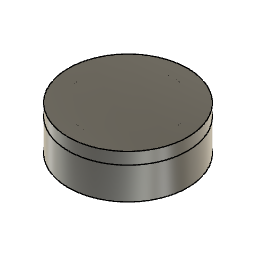
Zen_Garden_Model (Autodesk Fusion 360 design; units mm, degrees)
Autodesk Fusion 360 part; units mm, degrees
sketch "Sketch1" plane through (0, 0, 0) normal (0, 0, 1) x (1, 0, 0)
sketch "Sketch1 (2)" plane through (0, 0, 0) normal (0, 0, 1) x (1, 0, 0) in component "Base"
  circle A0 centre (0, 0) radius 120
  dimension "d2" = 240
  constraint coincident A0.centre origin
  measures "d2" diameter of A0
extrude "Extrude1" add sketch "Sketch1 (2)" along normal blind 10 makes body 1 in component "Base"
sketch "Sketch2" plane through (0, 0, 10) normal (0, 0, 1) x (-1, 0, 0) in component "Base"
  circle A0 centre (0, 0) radius 120
  circle A1 centre (0, 0) radius 100
  dimension "d5" = 20
  constraint coincident A0.centre A1.centre
  measures "d5" distance of A0 A1
extrude "Extrude2" add sketch "Sketch2" along normal blind 55 bodies 1 in component "Base"
sketch "Sketch3" plane through (0, 0, 65) normal (0, 0, 1) x (-1, 0, 0) in component "Base"
  circle A0 centre (0, 0) radius 100
  circle A1 centre (0, 0) radius 120
  circle A2 centre (0, 0) radius 107
  dimension "d10" = 7
  constraint coincident A0.centre A1.centre
  measures "d10" distance of A0 A2
extrude "Extrude3" add sketch "Sketch3" along normal blind 7 contours A1 bodies 1 in component "Base"
sketch "Sketch1 (3)" plane through (0, 0, 65) normal (0, 0, 1) x (-1, 0, 0) in component "Crown gear"
  circle A0 centre (0, 0) radius 73
  circle A1 centre (0, 0) radius 107
  circle A2 centre (0, 0) radius 107
  circle A3 centre (0, 0) radius 90 construction
  circle A4 centre (0, 0) radius 80
  circle A5 centre (0, 0) radius 100
  dimension "d92" = 180
  dimension "d164" = 7
  dimension "d168" = 7
  dimension "d170" = 10
  dimension "d171" = 10
  constraint coincident A0.centre A1.centre
  constraint equal A1 A2
  constraint concentric A2 A3
  constraint concentric A1 A4
  constraint concentric A1 A5
  measures "d92" diameter of A3
  measures "d164" distance of A1 A5
  measures "d168" distance of A0 A4
  measures "d170" distance of A3 A5
  measures "d171" distance of A3 A4
extrude "Extrude5" add sketch "Sketch1 (3)" against normal blind 15 separate body contours A1 A2 | A4 | A5 makes body 2 in component "Crown gear"
ref_plane "WorkPlane2" through (107, 0, 58.3628) normal (1, 0, 0) x (0, 1, 0) in component "Crown gear"
sketch "Sketch5" plane through (107, 0, 0) normal (1, 0, 0) x (0, 1, 0) in component "Crown gear"
  line L0 (-0.4478, 54) -> (-25.4478, 54) construction
  line L1 (-6.4157, 50) -> (-7.8716, 54)
  line L2 (-7.8716, 54) -> (-9.6915, 59)
  line L3 (-9.6915, 59) -> (0, 59)
  line L4 (0, 59) -> (-1.8199, 54)
  line L5 (-3.2757, 50) -> (-6.4157, 50)
  line L6 (-107, 50) -> (107, 50) construction
  line L7 (107, 65) -> (-107, 65) construction
  line L8 (-3.2757, 50) -> (-1.8199, 54)
  line L9 (0, 50) -> (0, 65) construction
  line L10 (3.2757, 50) -> (6.4157, 50)
  line L11 (6.4157, 50) -> (7.8716, 54)
  line L12 (0, 59) -> (1.8199, 54)
  line L13 (7.8716, 54) -> (9.6915, 59)
  line L14 (9.6915, 59) -> (0, 59)
  line L15 (3.2757, 50) -> (1.8199, 54)
  line L16 (3.2757, 50) -> (-3.2757, 50)
  point P0 (0, 50)
  point P1 (0.4478, 54)
  dimension "d102" = 70
  dimension "d103" = 70
  dimension "d104" = 4
  dimension "d105" = 5
  dimension "d107" = 3.14
  constraint horizontal L0
  constraint parallel L1 L2
  constraint parallel L0 L3
  constraint coincident L0 L4.end
  constraint horizontal L5
  constraint coincident L1.start L6
  constraint horizontal L0.start L1.end
  constraint equal L1 L8
  constraint midpoint L6 P0
  constraint midpoint L7 L9.end
  constraint vertical L3.end P0
  constraint symmetric L0.start L9 P1
  constraint symmetric L1.start L9 L10.end
  constraint symmetric L1.end L9 L11.end
  constraint symmetric L2.end L9 L13.end
  constraint symmetric L3.end L9 L4.start
  constraint symmetric L4.end L9 L12.end
  constraint symmetric L5.start L9 L10.start
  constraint symmetric P0 L9 L9.start
  measures "d102" angle of L0 L4
  measures "d103" angle of L0 L2
  measures "d104" vertical distance of L1.start L1.end
  measures "d105" vertical distance of L3.end L4.end
  measures "d107" distance of L1.start L5.start
extrude "Extrude6" cut sketch "Sketch5" along normal up to surface contours L4 L8 L12 L15 L16 end surface at (-72.6372, 7.2685, 55) on bodies 2 bodies 2 in component "Crown gear"
pattern_circular "C-Pattern2" count 45 over 360 about axis through (0, 0, 1.75) along (0, 0, 1) of "Extrude6" in component "Crown gear"
sketch "Sketch1 (4)" plane through (0, 0, 0) normal (1, 0, 0) x (0, 1, 0) in component "Pinion"
  circle A0 centre (0, 0) radius 20 construction
  circle A1 centre (0, 0) radius 20 construction
  circle A2 centre (0, 0) radius 18.7939
  circle A3 centre (0, 0) radius 24
  circle A4 centre (0, 0) radius 15
  line L0 (-18.7939, 0) -> (-18.7939, 29.5206) construction
  line L1 (0, 0) -> (-18.7939, 0) construction
  line L2 (0, 0) -> (-16.276, 9.3969) construction
  line L3 (0, 0) -> (-9.3969, 16.276) construction
  line L4 (0, 0) -> (0, 18.7939) construction
  line L5 (-16.276, 9.3969) -> (-6.4358, 26.4406) construction
  line L6 (-9.3969, 16.276) -> (-0.8751, 21.1961) construction
  spline S0 degree 5 poles (0, 18.7939) (0.0298, 18.9066) (0.0619, 19.1437) (0.0272, 19.5336) (-0.1787, 20.1207) (-0.672, 20.9554) (-1.3671, 21.8756) (-2.2385, 22.8636) (-3.2706, 23.8992) (-4.4543, 24.9586) (-5.7848, 26.0128) (-7.2591, 27.0265) (-8.8723, 27.9564) (-10.6168, 28.7521) (-12.485, 29.3613) (-14.4696, 29.7332) (-16.1459, 29.8058) (-17.4513, 29.7195) (-18.3428, 29.5976) (-18.7939, 29.5206) knots 0 0 0 0 0 0 0.066667 0.133333 0.2 0.266667 0.333333 0.4 0.466667 0.533333 0.6 0.666667 0.733333 0.8 0.866667 0.933333 1 1 1 1 1 1
  line L7 (0, 0) -> (-11.0467, 15.2045) construction
  line L8 (0, 18.7939) -> (-11.0467, 15.2045) construction
  line L9 (0, 0) -> (-5.5234, 16.9992) construction
  line L10 (0, 18.7939) -> (-5.5234, 16.9992) construction
  line L11 (0, 0) -> (-2.7617, 17.8965) construction
  spline S1 degree 5 poles (-5.6654, 17.9196) (-5.7278, 18.0181) (-5.8299, 18.2345) (-5.9144, 18.6168) (-5.895, 19.2386) (-5.6762, 20.1832) (-5.2909, 21.2701) (-4.7578, 22.4748) (-4.0859, 23.7734) (-3.2767, 25.1404) (-2.3258, 26.5465) (-1.2257, 27.9576) (0.0321, 29.3305) (1.4556, 30.6151) (3.0532, 31.759) (4.8334, 32.7119) (6.4098, 33.2865) (7.6805, 33.5977) (8.5673, 33.7502) (9.0206, 33.8128) knots 0 0 0 0 0 0 0.066667 0.133333 0.2 0.266667 0.333333 0.4 0.466667 0.533333 0.6 0.666667 0.733333 0.8 0.866667 0.933333 1 1 1 1 1 1
  line L12 (-0.4419, 17.1231) -> (0.4419, 20.4646)
  line L13 (-15.9559, 30.0052) -> (-21.6318, 29.036)
  line L14 (-4.7405, 16.4598) -> (-6.5903, 19.3794)
  line L15 (6.1687, 33.4193) -> (11.8726, 34.2062)
  point P0 (-5.5552, 20.4738)
  point P1 (-1.8342, 27.1507)
  dimension "d122" = 40
  dimension "d123" = 37.5877
  dimension "d124" = 48
  dimension "d125" = 30
  dimension "d126" = 29.5206
  dimension "d128" = -90
  dimension "d129" = 19.6804
  dimension "d130" = 9.8402
  dimension "d131" = 36
  constraint concentric A0 A1
  constraint concentric A0 A2
  constraint vertical A0.centre A1.centre
  constraint concentric A1 A3
  constraint concentric A2 A4
  constraint coincident A2 L0.start
  constraint tangent A2 L0
  constraint vertical L0
  constraint coincident A0.centre A1.centre
  constraint tangent A2 L5
  constraint perpendicular L2 L5
  constraint tangent A2 L6
  constraint perpendicular L3 L6
  constraint coincident A2 L7.end
  constraint midpoint L8 L9.end
  constraint midpoint L10 L11.end
  constraint midpoint L4.end L12
  constraint midpoint L0.end L13
  constraint symmetric L0.end L11 S1.end
  constraint symmetric L4.end L11 S1.start
  constraint symmetric L5.end L11 P1
  constraint symmetric L6.end L11 P0
  constraint symmetric L11 L12.start L14.start
  constraint symmetric L11 L12.end L14.end
  constraint symmetric L11 L13.start L15.start
  constraint symmetric L11 L13.end L15.end
  measures "d122" diameter of A0
  measures "d123" diameter of A2
  measures "d124" diameter of A3
  measures "d125" diameter of A4
  measures "d126" distance of L0.start L0.end
  measures "d129" distance of L2.end L5.end
  measures "d130" distance of L3.end L6.end
  measures "d131" angle of L4 L7
extrude "Extrude1'" add sketch "Sketch1 (4)" against normal blind 4 separate body contours A2 A3 S0 S1 picked at (-2.921, 21.0246) makes body 3 in component "Pinion"
pattern_circular "C-Pattern1" count 10 over 360 about axis through (1.75, 0, 0) along (1, 0, 0) of "Extrude1'" makes body 4 at (-0.3509, -16.7988, 14.2591) makes body 5 at (-0.3509, -21.9731, 1.6629) makes body 6 at (-0.3509, -18.755, -11.5701) makes body 7 at (-0.3509, -8.3701, -20.3829) makes body 8 at (-0.3509, 5.2072, -21.4147) makes body 9 at (-0.3509, 16.7988, -14.2591) makes body 10 at (-0.3509, 21.9731, -1.6629) makes body 11 at (-0.3509, 18.755, 11.5701) makes body 12 at (-0.3509, 8.3701, 20.3829) in component "Pinion"
extrude "Extrude2'" add sketch "Sketch1 (4)" against normal up to surface (4 mm away) contours A2 | A4 bodies 3 4 5 6 7 8 9 10 11 12 in component "Pinion"
sketch "Sketch8" plane through (0, 0, 0) normal (1, 0, 0) x (0, 1, 0) in component "Crown gear"
  line L0 (73, 59) -> (83, 59)
  line L1 (83, 59) -> (83, 50)
  line L2 (83, 50) -> (73, 50)
  line L3 (73, 50) -> (73, 59)
  line L4 (90, 65) -> (90, 50) construction
  line L5 (73, 65) -> (107, 65) construction
  line L6 (107, 50) -> (107, 59)
  line L7 (97, 50) -> (107, 50)
  line L8 (97, 59) -> (97, 50)
  line L9 (107, 59) -> (97, 59)
  point P0 (-73, 65)
  point P1 (73, 65)
  point P2 (107, 65)
  point P3 (-107, 65)
  point P4 (105.0137, 35)
  dimension "d139" = 9
  dimension "d140" = 10
  dimension "d172" = 6
  constraint horizontal L0
  constraint vertical L1
  constraint horizontal L2
  constraint vertical L3
  constraint vertical L4
  constraint coincident P1 L5.start
  constraint coincident P2 L5.end
  constraint midpoint L4.start L5
  constraint symmetric L0.start L4 L6.end
  constraint symmetric L0.end L4 L8.start
  constraint symmetric L1.end L4 L7.start
  constraint symmetric L4 L6.start L2.end
  constraint vertical P2 L6.start
  measures "d139" distance of L0.end L1.end
  measures "d140" distance of L0.start L0.end
  measures "d172" vertical distance of L0.start L5.start
revolve "Revolve2" cut sketch "Sketch8" angle 360 about axis through (0, 0, 1.75) along (0, 0, 1) bodies 2 in component "Crown gear"
sketch "Sketch2 (2)" plane through (0, 0, 0) normal (1, 0, 0) x (0, 1, 0) in component "Pinion"
  spline S0 degree 5 poles (17.874, 5.8076) (17.9905, 5.8141) (18.2258, 5.8569) (18.586, 6.0103) (19.0807, 6.3876) (19.7221, 7.1147) (20.3676, 8.0389) (20.8886, 8.9165) (21.274, 9.6386) (21.523, 10.1387) (21.6393, 10.3799) knots 0 0 0 0 0 0 0.066667 0.133333 0.2 0.266667 0.333333 0.392502 0.392502 0.392502 0.392502 0.392502 0.392502
  arc A0 (21.6393, 10.3799) -> (21.2067, 11.2372) centre (0, 0) ccw
  spline S1 degree 5 poles (15.2918, 10.9256) (15.3663, 11.0154) (15.5405, 11.1793) (15.878, 11.3778) (16.4753, 11.5516) (17.4413, 11.6354) (18.5681, 11.6054) (19.5836, 11.503) (20.3934, 11.3839) (20.9437, 11.2871) (21.2067, 11.2372) knots 0 0 0 0 0 0 0.066667 0.133333 0.2 0.266667 0.333333 0.392502 0.392502 0.392502 0.392502 0.392502 0.392502
  arc A1 (15.2918, 10.9256) -> (11.0467, 15.2045) centre (0, 0) ccw
  spline S2 degree 5 poles (11.0467, 15.2045) (11.1372, 15.2782) (11.3024, 15.4512) (11.5036, 15.787) (11.6821, 16.383) (11.7736, 17.3483) (11.7526, 18.4753) (11.6582, 19.4916) (11.5456, 20.3023) (11.4531, 20.8533) (11.4054, 21.1168) knots 0 0 0 0 0 0 0.066667 0.133333 0.2 0.266667 0.333333 0.392502 0.392502 0.392502 0.392502 0.392502 0.392502
  arc A2 (11.4054, 21.1168) -> (10.5515, 21.5561) centre (0, 0) ccw
  spline S3 degree 5 poles (5.9495, 17.8273) (5.9569, 17.9437) (6.0015, 18.1787) (6.1578, 18.5377) (6.539, 19.0294) (7.2712, 19.665) (8.2004, 20.3031) (9.0822, 20.8171) (9.8073, 21.1967) (10.3094, 21.4418) (10.5515, 21.5561) knots 0 0 0 0 0 0 0.066667 0.133333 0.2 0.266667 0.333333 0.392502 0.392502 0.392502 0.392502 0.392502 0.392502
  arc A3 (5.9495, 17.8273) -> (0, 18.7939) centre (0, 0) ccw
  spline S4 degree 5 poles (0, 18.7939) (0.0298, 18.9066) (0.0619, 19.1437) (0.0272, 19.5336) (-0.1787, 20.1207) (-0.672, 20.9554) (-1.3515, 21.8549) (-2.0252, 22.6216) (-2.5928, 23.2112) (-2.9915, 23.6027) (-3.185, 23.7877) knots 0 0 0 0 0 0 0.066667 0.133333 0.2 0.266667 0.333333 0.392502 0.392502 0.392502 0.392502 0.392502 0.392502
  arc A4 (-3.185, 23.7877) -> (-4.134, 23.6413) centre (0, 0) ccw
  spline S5 degree 5 poles (-5.6654, 17.9196) (-5.7278, 18.0181) (-5.8299, 18.2345) (-5.9144, 18.6168) (-5.895, 19.2386) (-5.6762, 20.1832) (-5.2995, 21.2456) (-4.8883, 22.1798) (-4.5249, 22.9131) (-4.2627, 23.4065) (-4.134, 23.6413) knots 0 0 0 0 0 0 0.066667 0.133333 0.2 0.266667 0.333333 0.392502 0.392502 0.392502 0.392502 0.392502 0.392502
  arc A5 (-5.6654, 17.9196) -> (-11.0467, 15.2045) centre (0, 0) ccw
  spline S6 degree 5 poles (-11.0467, 15.2045) (-11.0889, 15.3133) (-11.2023, 15.5239) (-11.4596, 15.8191) (-11.9712, 16.173) (-12.861, 16.5583) (-13.9393, 16.8866) (-14.935, 17.1109) (-15.7408, 17.2543) (-16.2935, 17.3366) (-16.5588, 17.3726) knots 0 0 0 0 0 0 0.066667 0.133333 0.2 0.266667 0.333333 0.392502 0.392502 0.392502 0.392502 0.392502 0.392502
  arc A6 (-16.5588, 17.3726) -> (-17.2405, 16.6963) centre (0, 0) ccw
  spline S7 degree 5 poles (-15.1163, 11.1672) (-15.2247, 11.2102) (-15.4344, 11.3253) (-15.7275, 11.5849) (-16.0774, 12.0994) (-16.4556, 12.9921) (-16.7753, 14.0731) (-16.9917, 15.0705) (-17.1287, 15.8774) (-17.2066, 16.4307) (-17.2405, 16.6963) knots 0 0 0 0 0 0 0.066667 0.133333 0.2 0.266667 0.333333 0.392502 0.392502 0.392502 0.392502 0.392502 0.392502
  arc A7 (-15.1163, 11.1672) -> (-17.874, 5.8076) centre (0, 0) ccw
  spline S8 degree 5 poles (-17.874, 5.8076) (-17.9721, 5.8708) (-18.1876, 5.9746) (-18.5692, 6.0621) (-19.1912, 6.0477) (-20.1375, 5.8364) (-21.2028, 5.4682) (-22.1402, 5.0644) (-22.8764, 4.7068) (-23.3719, 4.4485) (-23.6077, 4.3217) knots 0 0 0 0 0 0 0.066667 0.133333 0.2 0.266667 0.333333 0.392502 0.392502 0.392502 0.392502 0.392502 0.392502
  arc A8 (-23.6077, 4.3217) -> (-23.7617, 3.3739) centre (0, 0) ccw
  spline S9 degree 5 poles (-18.7933, 0.1493) (-18.9063, 0.1204) (-19.1435, 0.0902) (-19.5332, 0.128) (-20.1187, 0.3386) (-20.9494, 0.8385) (-21.8434, 1.5251) (-22.6048, 2.2049) (-23.1899, 2.7771) (-23.5781, 3.1789) (-23.7617, 3.3739) knots 0 0 0 0 0 0 0.066667 0.133333 0.2 0.266667 0.333333 0.392502 0.392502 0.392502 0.392502 0.392502 0.392502
  arc A9 (-18.7933, 0.1493) -> (-17.874, -5.8076) centre (0, 0) ccw
  spline S10 degree 5 poles (-17.874, -5.8076) (-17.9905, -5.8141) (-18.2258, -5.8569) (-18.586, -6.0103) (-19.0807, -6.3876) (-19.7221, -7.1147) (-20.3676, -8.0389) (-20.8886, -8.9165) (-21.274, -9.6386) (-21.523, -10.1387) (-21.6393, -10.3799) knots 0 0 0 0 0 0 0.066667 0.133333 0.2 0.266667 0.333333 0.392502 0.392502 0.392502 0.392502 0.392502 0.392502
  arc A10 (-21.6393, -10.3799) -> (-21.2067, -11.2372) centre (0, 0) ccw
  spline S11 degree 5 poles (-15.2918, -10.9256) (-15.3663, -11.0154) (-15.5405, -11.1793) (-15.878, -11.3778) (-16.4753, -11.5516) (-17.4413, -11.6354) (-18.5681, -11.6054) (-19.5836, -11.503) (-20.3934, -11.3839) (-20.9437, -11.2871) (-21.2067, -11.2372) knots 0 0 0 0 0 0 0.066667 0.133333 0.2 0.266667 0.333333 0.392502 0.392502 0.392502 0.392502 0.392502 0.392502
  arc A11 (-15.2918, -10.9256) -> (-11.0467, -15.2045) centre (0, 0) ccw
  spline S12 degree 5 poles (-11.0467, -15.2045) (-11.1372, -15.2782) (-11.3024, -15.4512) (-11.5036, -15.787) (-11.6821, -16.383) (-11.7736, -17.3483) (-11.7526, -18.4753) (-11.6582, -19.4916) (-11.5456, -20.3023) (-11.4531, -20.8533) (-11.4054, -21.1168) knots 0 0 0 0 0 0 0.066667 0.133333 0.2 0.266667 0.333333 0.392502 0.392502 0.392502 0.392502 0.392502 0.392502
  arc A12 (-11.4054, -21.1168) -> (-10.5515, -21.5561) centre (0, 0) ccw
  spline S13 degree 5 poles (-5.9495, -17.8273) (-5.9569, -17.9437) (-6.0015, -18.1787) (-6.1578, -18.5377) (-6.539, -19.0294) (-7.2712, -19.665) (-8.2004, -20.3031) (-9.0822, -20.8171) (-9.8073, -21.1967) (-10.3094, -21.4418) (-10.5515, -21.5561) knots 0 0 0 0 0 0 0.066667 0.133333 0.2 0.266667 0.333333 0.392502 0.392502 0.392502 0.392502 0.392502 0.392502
  arc A13 (-5.9495, -17.8273) -> (0, -18.7939) centre (0, 0) ccw
  spline S14 degree 5 poles (0, -18.7939) (-0.0298, -18.9066) (-0.0619, -19.1437) (-0.0272, -19.5336) (0.1787, -20.1207) (0.672, -20.9554) (1.3515, -21.8549) (2.0252, -22.6216) (2.5928, -23.2112) (2.9915, -23.6027) (3.185, -23.7877) knots 0 0 0 0 0 0 0.066667 0.133333 0.2 0.266667 0.333333 0.392502 0.392502 0.392502 0.392502 0.392502 0.392502
  arc A14 (3.185, -23.7877) -> (4.134, -23.6413) centre (0, 0) ccw
  spline S15 degree 5 poles (5.6654, -17.9196) (5.7278, -18.0181) (5.8299, -18.2345) (5.9144, -18.6168) (5.895, -19.2386) (5.6762, -20.1832) (5.2995, -21.2456) (4.8883, -22.1798) (4.5249, -22.9131) (4.2627, -23.4065) (4.134, -23.6413) knots 0 0 0 0 0 0 0.066667 0.133333 0.2 0.266667 0.333333 0.392502 0.392502 0.392502 0.392502 0.392502 0.392502
  arc A15 (5.6654, -17.9196) -> (11.0467, -15.2045) centre (0, 0) ccw
  spline S16 degree 5 poles (11.0467, -15.2045) (11.0889, -15.3133) (11.2023, -15.5239) (11.4596, -15.8191) (11.9712, -16.173) (12.861, -16.5583) (13.9393, -16.8866) (14.935, -17.1109) (15.7408, -17.2543) (16.2935, -17.3366) (16.5588, -17.3726) knots 0 0 0 0 0 0 0.066667 0.133333 0.2 0.266667 0.333333 0.392502 0.392502 0.392502 0.392502 0.392502 0.392502
  arc A16 (16.5588, -17.3726) -> (17.2405, -16.6963) centre (0, 0) ccw
  spline S17 degree 5 poles (15.1163, -11.1672) (15.2247, -11.2102) (15.4344, -11.3253) (15.7275, -11.5849) (16.0774, -12.0994) (16.4556, -12.9921) (16.7753, -14.0731) (16.9917, -15.0705) (17.1287, -15.8774) (17.2066, -16.4307) (17.2405, -16.6963) knots 0 0 0 0 0 0 0.066667 0.133333 0.2 0.266667 0.333333 0.392502 0.392502 0.392502 0.392502 0.392502 0.392502
  arc A17 (15.1163, -11.1672) -> (17.874, -5.8076) centre (0, 0) ccw
  spline S18 degree 5 poles (17.874, -5.8076) (17.9721, -5.8708) (18.1876, -5.9746) (18.5692, -6.0621) (19.1912, -6.0477) (20.1375, -5.8364) (21.2028, -5.4682) (22.1402, -5.0644) (22.8764, -4.7068) (23.3719, -4.4485) (23.6077, -4.3217) knots 0 0 0 0 0 0 0.066667 0.133333 0.2 0.266667 0.333333 0.392502 0.392502 0.392502 0.392502 0.392502 0.392502
  arc A18 (23.6077, -4.3217) -> (23.7617, -3.3739) centre (0, 0) ccw
  spline S19 degree 5 poles (18.7933, -0.1493) (18.9063, -0.1204) (19.1435, -0.0902) (19.5332, -0.128) (20.1187, -0.3386) (20.9494, -0.8385) (21.8434, -1.5251) (22.6048, -2.2049) (23.1899, -2.7771) (23.5781, -3.1789) (23.7617, -3.3739) knots 0 0 0 0 0 0 0.066667 0.133333 0.2 0.266667 0.333333 0.392502 0.392502 0.392502 0.392502 0.392502 0.392502
  arc A19 (18.7933, -0.1493) -> (17.874, 5.8076) centre (0, 0) ccw
  circle A20 centre (0, 0) radius 1
  dimension "d147" = 2
  constraint coincident A0.centre A1.centre
  measures "d147" diameter of A20
extrude "Extrude3'" cut sketch "Sketch2 (2)" against normal up to surface (4 mm away) contours A20 bodies 3 in component "Pinion"
sketch "Sketch1 (5)" plane through (0, 0, 0) normal (0, 0, 1) x (1, 0, 0) in component "DcMotor"
  circle A0 centre (0, 0) radius 12.2
  dimension "d151" = 24.4
  constraint coincident A0.centre origin
  measures "d151" diameter of A0
extrude "Extrude1''" add sketch "Sketch1 (5)" along normal blind 12.8 separate body makes body 13 in component "DcMotor"
sketch "Sketch2 (3)" plane through (0, 0, 12.8) normal (0, 0, 1) x (-1, 0, 0) in component "DcMotor"
  circle A0 centre (0, 0) radius 12.2
  circle A1 centre (0, 0) radius 3.225
  dimension "d154" = 6.45
  constraint concentric A0 A1
  measures "d154" diameter of A1
extrude "Extrude2''" add sketch "Sketch2 (3)" along normal blind 1 contours A1 bodies 13 in component "DcMotor"
sketch "Sketch3 (2)" plane through (0, 0, 13.8) normal (0, 0, 1) x (-1, 0, 0) in component "DcMotor"
  circle A0 centre (0, 0) radius 3.225
  circle A1 centre (0, 0) radius 1
  dimension "d157" = 2
  constraint concentric A0 A1
  measures "d157" diameter of A1
extrude "Extrude3''" add sketch "Sketch3 (2)" along normal blind 6 contours A1 bodies 13 in component "DcMotor"
sketch "Sketch4" plane through (0, 0, 10) normal (0, 0, 1) x (-1, 0, 0) in component "Base"
  circle A0 centre (0, 0) radius 100
  circle A1 centre (0, 0) radius 15
  dimension "d177" = 30
  constraint concentric A0 A1
  measures "d177" diameter of A1
extrude "Extrude4" add sketch "Sketch4" along normal blind 20 contours A1 bodies 1 in component "Base"
sketch "Sketch5 (2)" plane through (0, 0, 30) normal (0, 0, 1) x (-1, 0, 0) in component "Base"
  circle A0 centre (0, 0) radius 15
  circle A1 centre (0, 0) radius 12.5
  dimension "d181" = 25
  constraint concentric A0 A1
  measures "d181" diameter of A1
extrude "Extrude5'" cut sketch "Sketch5 (2)" against normal blind 3 contours A1 bodies 1 in component "Base"
sketch "Sketch6" plane through (0, 0, 10) normal (0, 0, 1) x (-1, 0, 0) in component "Base"
  circle A0 centre (0, 0) radius 15
  circle A1 centre (0, 0) radius 100
  line L0 (-88, 15) -> (-68, 15)
  line L1 (-68, 15) -> (-68, -15)
  line L2 (-68, -15) -> (-88, -15)
  line L3 (-88, -15) -> (-88, 15)
  line L4 (-88, 0) -> (-68, 0) construction
  dimension "d188" = 30
  dimension "d189" = 20
  dimension "d191" = 68
  constraint horizontal L0
  constraint vertical L1
  constraint horizontal L2
  constraint vertical L3
  constraint midpoint L3 L4.start
  constraint midpoint L1 L4.end
  constraint horizontal A0.centre L4.end
  measures "d188" distance of L0.end L1.end
  measures "d189" distance of L0.start L0.end
  measures "d191" distance of A0.centre L1
extrude "Extrude6'" add sketch "Sketch6" along normal blind 44 contours L0 L1 L2 L3 bodies 1 in component "Base"
ref_plane "WorkPlane1" through (78, 0, 32) normal (-1, 0, 0) x (0, -1, 0) in component "Base"
sketch "Sketch8 (2)" plane through (78, 0, 0) normal (-1, 0, 0) x (0, -1, 0) in component "Base"
  circle A0 centre (0.0107, 37) radius 12.5
  line L0 (-15, 54) -> (15, 54)
  line L1 (-12.4893, 37) -> (-12.4893, 54)
  line L2 (12.505, 37.3751) -> (12.0059, 54)
  line L3 (-15, 10) -> (15, 10)
  dimension "d200" = 25
  dimension "d201" = 27
  constraint coincident A0 L1.start
  constraint coincident L0 L1.end
  constraint perpendicular L0 L1
  constraint tangent A0 L1
  constraint coincident A0 L2.start
  constraint coincident L0 L2.end
  constraint tangent A0 L2
  measures "d200" diameter of A0
  measures "d201" distance of A0.centre L3
extrude "Extrude8" cut sketch "Sketch8 (2)" along normal mid plane 16 bodies 1 in component "Base"
sketch "Sketch9" plane through (88, 0, 0) normal (1, 0, 0) x (0, 1, 0) in component "Base"
  line L0 (-15, 10) -> (15, 10)
  line L1 (15, 10) -> (15, 54)
  line L2 (15, 54) -> (-15, 54)
  line L3 (-15, 54) -> (-15, 10)
  line L4 (-10, 54) -> (10, 54)
  line L5 (10, 54) -> (10, 34)
  line L6 (10, 34) -> (-10, 34)
  line L7 (-10, 34) -> (-10, 54)
  dimension "d204" = 5
  dimension "d205" = 5
  dimension "d206" = 24
  constraint horizontal L4
  constraint vertical L5
  constraint horizontal L6
  constraint vertical L7
  constraint coincident L2 L4.start
  measures "d204" distance of L3 L7
  measures "d205" distance of L1 L5
  measures "d206" distance of L0.start L6
extrude "Extrude9" cut sketch "Sketch9" against normal up to surface (2 mm away) contours L2 L4 L5 L6 L7 bodies 1 in component "Base"
component "Base" placed x (1, 0, 0) y (0, 1, 0) z (0, 0, 1) at (0, 0, 0)
component "Crown gear" placed x (-0.234021, 0.972232, 0) y (-0.972232, -0.234021, 0) z (0, 0, 1) at (0, 0, 6)
component "Pinion" placed x (-1, 0, 0) y (0, 0.905578, -0.42418) z (0, -0.42418, -0.905578) at (87.4, -0.0107, 37)
component "DcMotor" placed x (0, 0, 1) y (0, -1, 0) z (1, 0, 0) at (71.6, -0.0107, 37)
component "DcMotor" placed x (-1, 0, 0) y (0, -1, 0) z (0, 0, 1) at (0, 0, 27)
equation "radious = 120 mm" comment "Base diameter"
equation "d2 = radious * 2"
equation "d5 = thickness"
equation "d6 = motor_heigth"
equation "motor_heigth = 55 mm" comment "Motor spacing from the base to the gear's teeth"
equation "d10 = padding_gear"
equation "d11 = crow_thickness - ( 2.25 * module ) + 1 mm"
equation "thickness = 20 mm" comment "Border thickness of the base"
equation "padding_gear = 7 mm" comment "The space to hold the crown in its position"
equation "d92 = pitch_diameter1"
equation "module = 4 mm" comment "Module gear"
equation "zp = ( 10 mm ) / mm" comment "Pinion teeth number"
equation "zc = pitch_diameter1 / module" comment "Gear teeth number"
equation "pitch_diameter1 = 180 mm" comment "The principal diameter of the face gear"
equation "crow_thickness = 15 mm" comment "The thickness of the gear from the teeth to the base of the crown."
equation "d98 = -crow_thickness"
equation "d103 = d102"
equation "d104 = module * 1"
equation "d105 = 1.25 * module"
equation "d110 = zc"
equation "d116 = padding_gear"
equation "d122 = module * zp"
equation "d123 = d122 * cos(20 deg)"
equation "d124 = d122 + 2 * module"
equation "d125 = d122 - 2 * ( 1.25 * module )"
equation "d126 = ( d123 * 3.141516 ) / 4"
equation "d129 = d126 * 2 / 3"
equation "d130 = d126 / 3"
equation "d131 = ( 360 / zp ) * 1 deg"
equation "d134 = zp"
equation "d139 = 2.25 * module"
equation "d140 = padding_gear + 3 mm"
equation "d147 = motor_axis_diameter"
equation "motor_axis_diameter = 2 mm"
equation "d164 = padding_gear"
equation "d168 = padding_gear"
equation "d171 = d170"
equation "d172 = crow_thickness - d139"
equation "motor_offset = 20 mm"
equation "d179 = motor_offset"
equation "axis_to_angle_motor = radious - thickness - 32 mm"
equation "d191 = axis_to_angle_motor"
equation "d192 = motor_heigth - module * 2.25 - 2 mm"
equation "d205 = d204"
equation "d219 = ( -36 * 45 ) * 1 deg"
